Autodesk Fusion 360 part; units mm, degrees
note: some values were not read from the file. Chosen so that the rebuilt part matches the saved one: which bodies a step acts on. Set by a fixed rule: which sketch regions a step uses.
(part 2 of 2)
sketch "Sketch22" plane through (160, 0, 0) normal (1, 0, 0) x (0, 1, 0)
  line L0 (15.6749, -37) -> (15.6749, 8)
  line L1 (15.6749, 8) -> (-86.3257, 8)
  line L2 (-86.3257, 8) -> (-86.3257, -37)
  line L3 (-86.3257, -37) -> (15.6749, -37)
  line L4 (12.6241, -34) -> (12.6713, 4.9905)
  line L5 (4.6205, -36.9903) -> (4.6241, -33.9903)
  line L6 (4.6241, -33.9903) -> (12.6241, -34)
  line L7 (4.6205, -36.9903) -> (-15.3795, -36.9661)
  line L8 (-15.3795, -36.9661) -> (-15.3758, -33.9661)
  line L9 (-15.3758, -33.9661) -> (-25.3758, -33.9541)
  line L10 (-25.3758, -33.9541) -> (-25.3758, -36.9541)
  line L11 (-25.3758, -36.9541) -> (-45.3758, -36.9541)
  line L12 (-45.3758, -36.9541) -> (-45.3758, -33.9541)
  line L13 (-45.3758, -33.9541) -> (-55.3758, -33.9541)
  line L14 (-55.3758, -33.9541) -> (-55.3758, -36.9541)
  line L15 (-75.3758, -36.9541) -> (-75.3758, -33.9541)
  line L16 (-75.3758, -33.9541) -> (-83.3257, -33.9541)
  line L17 (-25.3817, 8) -> (-25.2839, 8)
  line L18 (-15.3817, 8) -> (-15.3817, 8.0002)
  line L19 (4.6183, 8.0002) -> (4.6183, 8)
  line L20 (-75.3758, -36.9541) -> (-55.3758, -36.9541)
  line L21 (-83.3257, -33.9541) -> (-83.3257, 8.0459)
  line L22 (-83.3257, 8.0459) -> (-75.3257, 8.0459)
  line L23 (-75.3257, 8.0459) -> (-75.3257, 11.0459)
  line L24 (-75.3257, 11.0459) -> (-55.3257, 11.0459)
  line L25 (-55.3257, 11.0459) -> (-55.3257, 8.0459)
  line L26 (-55.3257, 8.0459) -> (-45.3257, 8.0459)
  line L27 (-45.3257, 8.0459) -> (-45.3257, 11.0459)
  line L28 (-45.3257, 11.0459) -> (-25.3257, 11.0459)
  line L29 (-25.3257, 11.0459) -> (-25.3257, 8.0459)
  line L30 (-25.3257, 8.0459) -> (-15.3257, 8.0459)
  line L31 (-15.3257, 8.0459) -> (-15.3257, 11.0459)
  line L32 (-15.3257, 11.0459) -> (4.6743, 11.0459)
  line L33 (4.6743, 11.0459) -> (4.6743, 8.0459)
  line L34 (4.6743, 8.0459) -> (12.6743, 8.0459)
  line L35 (12.6743, 8.0459) -> (12.6713, 4.9905)
  line L36 (12.6743, 8.0459) -> (12.6743, 0.0459)
  line L37 (12.6743, 0.0459) -> (12.6653, 0.0459)
  line L38 (4.6743, 0.0459) -> (4.6743, -2.9541)
  line L39 (4.6743, -2.9541) -> (-15.3257, -2.9541)
  line L40 (-15.3257, -2.9541) -> (-15.3257, 0.0459)
  line L41 (-15.3257, 0.0459) -> (4.6743, 0.0459)
  line L42 (-25.3257, 0.0459) -> (-25.3257, -2.9541)
  line L43 (-25.3257, -2.9541) -> (-45.3257, -2.9541)
  line L44 (-45.3257, -2.9541) -> (-45.3257, 0.0459)
  line L45 (-45.3257, 0.0459) -> (-25.3257, 0.0459)
  line L46 (-55.3257, -2.9541) -> (-55.3257, 0.0459)
  line L47 (-55.3257, 0.0459) -> (-75.3257, 0.0459)
  line L48 (-75.3257, 0.0459) -> (-75.3257, -2.9541)
  line L49 (-75.3257, -2.9541) -> (-55.3257, -2.9541)
  point P0 (4.6746, -55)
  point P1 (-15.3254, -55)
  point P2 (-25.3254, -55)
  point P3 (-45.3254, -55)
  point P4 (-55.3254, -55)
  point P5 (-75.3254, -55)
  dimension "d176" = 3
  dimension "d177" = 20
  dimension "d178" = 3
  dimension "d179" = 10
  dimension "d180" = 3
  dimension "d181" = 20
  dimension "d182" = 3
  dimension "d183" = 10
  dimension "d184" = 20
  dimension "d185" = 3
  dimension "d194" = 20
  dimension "d196" = 42
  dimension "d197" = 8
  dimension "d198" = 3
  dimension "d199" = 20
  dimension "d200" = 3
  dimension "d201" = 10
  dimension "d202" = 20
  dimension "d203" = 3
  dimension "d204" = 10
  dimension "d205" = 20
  dimension "d206" = 3
  dimension "d207" = 8
  dimension "d208" = 8
  dimension "d209" = 8
  dimension "d210" = 3
  dimension "d211" = 20
  dimension "d212" = 10
  dimension "d213" = 3
  dimension "d214" = 20
  dimension "d215" = 10
  dimension "d216" = 20
  dimension "d217" = 3
  constraint perpendicular L4 L6
  constraint perpendicular L5 L7
  constraint perpendicular L7 L8
  constraint perpendicular L8 L9
  constraint perpendicular L3 L10
  constraint perpendicular L10 L11
  constraint perpendicular L11 L12
  constraint perpendicular L12 L13
  constraint perpendicular L13 L14
  constraint perpendicular L3 L15
  constraint coincident L1 L17.start
  constraint perpendicular L14 L20
  constraint coincident L1 L18.start
  constraint coincident L1 L19.end
  constraint perpendicular L1 L21
  constraint perpendicular L21 L22
  constraint perpendicular L22 L23
  constraint perpendicular L23 L24
  constraint perpendicular L1 L25
  constraint perpendicular L25 L26
  constraint perpendicular L1 L27
  constraint perpendicular L27 L28
  constraint perpendicular L1 L29
  constraint perpendicular L29 L30
  constraint perpendicular L1 L31
  constraint perpendicular L29 L32
  constraint perpendicular L1 L33
  constraint perpendicular L33 L34
  constraint perpendicular L1 L36
  constraint perpendicular L36 L37
  constraint perpendicular L37 L38
  constraint perpendicular L38 L39
  constraint perpendicular L39 L40
  constraint perpendicular L38 L41
  constraint perpendicular L42 L43
  constraint perpendicular L43 L44
  constraint perpendicular L42 L45
  constraint perpendicular L46 L47
  constraint perpendicular L47 L48
  constraint perpendicular L48 L49
  constraint coincident L4 L37.end
  measures "d176" distance of L5.start L5.end
  measures "d177" distance of L5.start L7.end
  measures "d178" distance of L7.end L8.end
  measures "d179" distance of L8.end L9.end
  measures "d180" distance of L9.end L10.end
  measures "d181" distance of L10.end L11.end
  measures "d182" distance of L11.end L12.end
  measures "d183" distance of L12.end L13.end
  measures "d184" distance of L14.end L15.start
  measures "d185" distance of L15.start L15.end
  measures "d194" distance of L18.end L19.start
  measures "d196" distance of L16.end L21.end
  measures "d197" distance of L21.end L22.end
  measures "d198" distance of L22.end L23.end
  measures "d199" distance of L23.end L24.end
  measures "d200" distance of L24.end L25.end
  measures "d201" distance of L25.end L26.end
  measures "d202" distance of L27.end L28.end
  measures "d203" distance of L28.end L29.end
  measures "d204" distance of L29.end L30.end
  measures "d205" distance of L31.end L32.end
  measures "d206" distance of L32.end L33.end
  measures "d207" distance of L33.end L34.end
  measures "d208" distance of L34.end L36.end
  measures "d209" distance of L36.end L38.start
  measures "d210" distance of L38.start L38.end
  measures "d211" distance of L38.end L39.end
  measures "d212" distance of L40.end L42.start
  measures "d213" distance of L42.start L42.end
  measures "d214" distance of L42.end L43.end
  measures "d215" distance of L43.end L46.start
  measures "d216" distance of L46.end L47.end
  measures "d217" distance of L47.end L48.end
ref_plane "WorkPlane7" through (203.1759, -36.8254, -17) normal (1, 0, 0) x (0, 0, -1)
sketch "Sketch23" plane through (203.1759, 0, 0) normal (1, 0, 0) x (0, 1, 0)
  line L0 (4.6241, -33.9903) -> (12.6241, -34)
  line L1 (4.6205, -36.9903) -> (4.6241, -33.9903)
  line L2 (4.6205, -36.9903) -> (-15.3795, -36.9661)
  line L3 (-15.3795, -36.9661) -> (-15.3758, -33.9661)
  line L4 (-15.3758, -33.9661) -> (-25.3758, -33.9541)
  line L5 (-25.3758, -33.9541) -> (-25.3758, -36.9541)
  line L6 (-25.3758, -36.9541) -> (-45.3758, -36.9541)
  line L7 (-45.3758, -36.9541) -> (-45.3758, -33.9541)
  line L8 (-45.3758, -33.9541) -> (-55.3758, -33.9541)
  line L9 (-55.3758, -33.9541) -> (-55.3758, -36.9541)
  line L10 (-75.3758, -36.9541) -> (-55.3758, -36.9541)
  line L11 (-75.3758, -36.9541) -> (-75.3758, -33.9541)
  line L12 (-75.3758, -33.9541) -> (-83.3257, -33.9541)
  line L13 (-75.3257, 0.0459) -> (-75.3257, -2.9541)
  line L14 (-75.3257, -2.9541) -> (-55.3257, -2.9541)
  line L15 (-55.3257, -2.9541) -> (-55.3257, 0.0459)
  line L16 (-45.3257, -2.9541) -> (-45.3257, 0.0459)
  line L17 (-25.3257, -2.9541) -> (-45.3257, -2.9541)
  line L18 (-25.3257, 0.0459) -> (-25.3257, -2.9541)
  line L19 (-15.3257, -2.9541) -> (-15.3257, 0.0459)
  line L20 (4.6743, -2.9541) -> (-15.3257, -2.9541)
  line L21 (4.6743, 0.0459) -> (4.6743, -2.9541)
  line L22 (4.6743, 0.0459) -> (12.6743, 0.0459)
  line L23 (12.6743, 0.0459) -> (12.6241, -34)
  line L24 (-15.3795, -36.9661) -> (4.6205, -36.9903)
  line L25 (-25.3758, -36.9541) -> (-45.3758, -36.9541)
  line L26 (-55.3758, -36.9541) -> (-75.3758, -36.9541)
  line L27 (-83.3257, -33.9541) -> (-83.3257, 0.0459)
  line L28 (-83.3257, 0.0459) -> (-75.3257, 0.0459)
  line L29 (-55.3257, 0.0459) -> (-45.3257, 0.0459)
  line L30 (-25.3257, 0.0459) -> (-15.3257, 0.0459)
  dimension "d219" = 8
  dimension "d220" = 34
  constraint coincident L21.start L22.start
  constraint perpendicular L21 L22
  constraint coincident L0.end L23.end
  constraint coincident L2.end L3.start
  constraint coincident L1.start L2.start
  constraint coincident L5.end L6.start
  constraint coincident L6.end L7.start
  constraint coincident L9.end L10.end
  constraint coincident L10.start L11.start
  constraint coincident L12.end L27.start
  constraint perpendicular L12 L27
  constraint coincident L13.start L28.end
  constraint coincident L15.end L29.start
  constraint coincident L16.end L29.end
  constraint coincident L18.start L30.start
  constraint coincident L19.end L30.end
  measures "d219" distance of L21.start L22.end
  measures "d220" distance of L12.end L27.end
ref_plane "WorkPlane8" through (29.5575, -36.8254, 55) normal (0, 0, 1) x (1, 0, 0)
sketch "Sketch24" plane through (0, 0, 55) normal (0, 0, 1) x (1, 0, 0)
  line L0 (60.1759, 4.6746) -> (63.1759, 4.6746)
  line L1 (63.1759, 4.6746) -> (63.1759, -15.3254)
  line L2 (60.1759, -15.3254) -> (63.1759, -15.3254)
  line L3 (60.1759, -25.3254) -> (63.1759, -25.3254)
  line L4 (63.1759, -25.3254) -> (63.1759, -45.3254)
  line L5 (60.1759, -45.3254) -> (63.1759, -45.3254)
  line L6 (60.1759, -55.3254) -> (63.1759, -55.3254)
  line L7 (63.1759, -55.3254) -> (63.1759, -75.3254)
  line L8 (60.1759, -75.3254) -> (63.1759, -75.3254)
  line L9 (-4.0608, -75.3254) -> (-7.0608, -75.3254)
  line L10 (-4.0608, -55.3254) -> (-7.0608, -55.3254)
  line L11 (-4.0608, -45.3254) -> (-7.0608, -45.3254)
  line L12 (-4.0608, -25.3254) -> (-7.0608, -25.3254)
  line L13 (-4.0608, -15.3254) -> (-7.0608, -15.3254)
  line L14 (-4.0608, 4.6746) -> (-7.0608, 4.6746)
  line L15 (60.1759, -75.3254) -> (60.1759, -83.3254)
  line L16 (-7.0608, -75.3254) -> (-7.0608, -55.3254)
  line L17 (-4.0608, -55.3254) -> (-4.0608, -45.3254)
  line L18 (-7.0608, -45.3254) -> (-7.0608, -25.3254)
  line L19 (-4.0608, -25.3254) -> (-4.0608, -15.3254)
  line L20 (-7.0608, -15.3254) -> (-7.0608, 4.6746)
  line L21 (-4.0608, 4.6746) -> (-4.0608, 12.6746)
  line L22 (-4.0608, 12.6746) -> (59.9392, 12.6746)
  line L23 (59.9392, 12.6746) -> (60.1759, 4.6746)
  line L24 (63.1759, 4.6746) -> (63.1759, -15.3254)
  line L25 (60.1759, -15.3254) -> (60.1759, -25.3254)
  line L26 (63.1759, -45.3254) -> (63.1759, -25.3254)
  line L27 (60.1759, -45.3254) -> (60.1759, -46.3367)
  line L28 (60.1759, -46.3367) -> (60.1759, -55.3254)
  line L29 (63.1759, -55.3254) -> (63.1759, -75.3254)
  circle A0 centre (5.08, -54.958) radius 1.75
  circle A1 centre (5.08, -15.08) radius 1.75
  line L30 (-4.0608, -75.3254) -> (-4.0608, -83.3254)
  line L31 (-4.0608, -83.3254) -> (60.1759, -83.3254)
  dimension "d224" = 8
  dimension "d225" = 64
  dimension "d243" = 8
  constraint coincident L8.start L15.start
  constraint perpendicular L8 L15
  constraint coincident L9.end L16.start
  constraint coincident L10.end L16.end
  constraint coincident L10.start L17.start
  constraint coincident L11.start L17.end
  constraint coincident L11.end L18.start
  constraint coincident L12.end L18.end
  constraint coincident L12.start L19.start
  constraint coincident L13.start L19.end
  constraint coincident L13.end L20.start
  constraint coincident L14.end L20.end
  constraint coincident L14.start L21.start
  constraint perpendicular L14 L21
  constraint perpendicular L21 L22
  constraint coincident L0.start L23.end
  constraint coincident L0.end L1.start
  constraint coincident L1.end L2.end
  constraint coincident L2.start L25.start
  constraint coincident L3.start L25.end
  constraint coincident L4.end L5.end
  constraint coincident L3.end L4.start
  constraint coincident L5.start L27.start
  constraint perpendicular L5 L27
  constraint coincident L6.start L28.end
  constraint perpendicular L6 L28
  constraint coincident L6.end L7.start
  constraint coincident L7.end L8.end
  constraint coincident L9.start L30.start
  constraint perpendicular L9 L30
  constraint perpendicular L15 L31
  measures "d224" distance of L14.start L21.end
  measures "d225" distance of L21.end L22.end
  measures "d243" distance of L9.start L30.end
sketch "nfc_haut" plane through (0, 0, 0) normal (0, 0, 1) x (1, 0, 0)
  line L0 (-7.0608, -86.3257) -> (134.0003, -86.3257)
  line L1 (134.0003, -86.3257) -> (134.0003, 15.6749)
  line L2 (-7.0608, 15.6749) -> (-7.0608, -86.3257)
  line L3 (134.0003, 15.6749) -> (-7.0608, 15.6749)
  circle A0 centre (95, 2.5) radius 1.5
  circle A1 centre (95, -72.5) radius 1.5
  circle A2 centre (126, -72.5) radius 1.5
  circle A3 centre (126, 2.5) radius 1.5
  line L4 (114.0003, -83.3257) -> (80.1759, -83.3257)
  line L5 (80.1759, -86.3257) -> (80.1759, -83.3257)
  line L6 (114.0003, -86.3257) -> (114.0003, -83.3257)
  line L7 (114.0003, 15.6749) -> (114.0003, 12.6749)
  line L8 (114.0003, 12.6749) -> (84.0003, 12.6749)
  line L9 (84.0003, 12.6749) -> (84.0003, 15.6749)
  line L10 (42.9392, 12.6749) -> (42.9392, 15.6749)
  line L11 (12.9392, 12.6749) -> (42.9392, 12.6749)
  line L12 (12.9392, 15.6749) -> (12.9392, 12.6749)
  line L13 (-4.0608, -5.3254) -> (-4.0608, 4.6746)
  line L14 (-4.0608, 4.6746) -> (-7.0608, 4.6746)
  line L15 (-4.0608, -5.3254) -> (-4.0608, -15.3254)
  line L16 (-4.0608, -15.3254) -> (-7.0608, -15.3254)
  line L17 (-4.0608, -25.3254) -> (-7.0608, -25.3254)
  line L18 (-4.0608, -35.3254) -> (-4.0608, -25.3254)
  line L19 (-4.0608, -35.3254) -> (-4.0608, -45.3254)
  line L20 (-4.0608, -45.3254) -> (-7.0608, -45.3254)
  line L21 (-4.0608, -55.3254) -> (-7.0608, -55.3254)
  line L22 (-4.0608, -65.3254) -> (-4.0608, -55.3254)
  line L23 (-4.0608, -65.3254) -> (-4.0608, -75.3254)
  line L24 (-4.0608, -75.3254) -> (-7.0608, -75.3254)
  line L25 (131.0003, -75.3254) -> (134.0003, -75.3254)
  line L26 (131.0003, -65.3254) -> (131.0003, -75.3254)
  line L27 (131.0003, -65.3254) -> (131.0003, -55.3254)
  line L28 (131.0003, -55.3254) -> (134.0003, -55.3254)
  line L29 (131.0003, -15.3254) -> (134.0003, -15.3254)
  line L30 (131.0003, -5.3254) -> (131.0003, -15.3254)
  line L31 (131.0003, -5.3254) -> (131.0003, 4.6746)
  line L32 (131.0003, 4.6746) -> (134.0003, 4.6746)
  line L33 (131.0003, -25.3254) -> (134.0003, -25.3254)
  line L34 (131.0003, -35.3254) -> (131.0003, -25.3254)
  line L35 (131.0003, -35.3254) -> (131.0003, -45.3254)
  line L36 (131.0003, -45.3254) -> (134.0003, -45.3254)
  line L37 (60.1759, 4.6746) -> (63.1759, 4.6746)
  line L38 (63.1759, -15.3254) -> (60.1759, -15.3254)
  line L39 (60.1759, -15.3254) -> (60.1759, 4.6746)
  line L40 (63.1759, 4.6746) -> (63.1759, -15.3254)
  line L41 (60.1759, -45.3254) -> (60.1759, -25.3254)
  line L42 (63.1759, -45.3254) -> (60.1759, -45.3254)
  line L43 (60.1759, -25.3254) -> (63.1759, -25.3254)
  line L44 (63.1759, -25.3254) -> (63.1759, -45.3254)
  line L45 (63.1759, -75.3254) -> (60.1759, -75.3254)
  line L46 (63.1759, -55.3254) -> (63.1759, -75.3254)
  line L47 (60.1759, -75.3254) -> (60.1759, -55.3254)
  line L48 (60.1759, -55.3254) -> (63.1759, -55.3254)
  line L49 (12.9392, -86.3257) -> (12.9392, -83.3257)
  line L50 (12.9392, -83.3257) -> (42.9392, -83.3257)
  line L51 (42.9392, -83.3257) -> (42.9392, -86.3257)
  line L52 (123.5599, -71.6605) -> (96.4401, -71.6605)
  line L53 (96.4401, -71.6605) -> (96.4401, 1.6605)
  line L54 (96.4401, 1.6605) -> (123.5599, 1.6605)
  line L55 (123.5599, 1.6605) -> (123.5599, -71.6605)
  constraint horizontal L52
  constraint perpendicular L52 L53
  constraint parallel L52 L54
  constraint parallel L53 L55
hidden bodies 1
equation "larg_LCD = 36 mm"
equation "Long_lcd = 80 mm"
equation "Trou_lcd = 2.5 mm"
equation "diam_trou_lcd = 4 mm"
equation "d5 = Long_lcd"
equation "d6 = larg_LCD"
named bodies: "LCD", "Cartelecteur"
